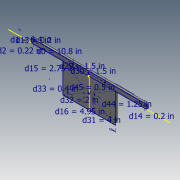
# Autodesk Inventor part: VP TRAY PUSHER TOP
Saved by Autodesk Inventor 2018.3 (Build 223284000, 284)
## iProperties
Created: 2019-10-29
Material: Generic
Vendor: HHMI: JRC - ID&F
Document SubType Name: Modeling
Designer: arnoldj
Density: 1 g/cm^3
Appearance: Default
RuleStatus: InUse
AfterDocSave0: file://Part Number Cleaner
DESIGN DEPARTMENT: HHMI: JRC - ID&F
ALTERED ITEM PART NUMBER: N/A
ALTERED ITEM VENDOR: N/A
ALTERED ITEM DESCRIPTION: N/A
Author: arnoldj
Revision Number: 0
Autodesk Inventor part; units mm, degrees
ref_plane "YZ Plane" through (0, 0, 0) normal (1, 0, 0) x (0, 1, 0)
ref_plane "XZ Plane" through (0, 0, 0) normal (0, 1, 0) x (-1, 0, 0)
ref_plane "XY Plane" through (0, 0, 0) normal (0, 0, 1) x (1, 0, 0)
sketch "Sketch1" plane through (0, 0, 0) normal (0, 0, 1) x (1, 0, 0)
  line L0 (0, 26.162) -> (0, -85.852) projected
  line L1 (-192.024, 0) -> (192.024, 0) projected
  line L2 (137.16, 10.16) -> (-137.16, 10.16)
  line L3 (-137.16, 10.16) -> (-137.16, 0)
  line L4 (-137.16, 0) -> (137.16, 0)
  line L5 (137.16, 0) -> (137.16, 10.16)
  line L6 (137.16, 10.16) -> (-137.16, 0) construction
  line L7 (-137.16, 10.16) -> (137.16, 0) construction
  line L8 (62.865, -69.85) -> (-62.865, -69.85)
  line L9 (-62.865, -69.85) -> (-62.865, 0)
  line L10 (-62.865, 0) -> (62.865, 0)
  line L11 (62.865, 0) -> (62.865, -69.85)
  line L12 (62.865, -69.85) -> (-62.865, 0) construction
  line L13 (-62.865, -69.85) -> (62.865, 0) construction
  point P0 (0, 0)
  point P1 (0, 5.08)
  point P2 (0, 5.588)
  point P3 (-132.08, 5.588)
  point P4 (132.08, 5.588)
  point P5 (0, -34.925)
  point P6 (12.7, -31.75)
  point P7 (-38.1, 5.588)
  point P8 (38.1, 5.588)
  point P9 (-50.8, -59.69)
  point P10 (50.8, -59.69)
  point P11 (0, -34.925)
  dimension "d0" = 274.32
  dimension "d1" = 10.16
  dimension "d2" = 5.588
  dimension "d13" = 5.08
  dimension "d14" = 5.08
  dimension "d15" = 69.85
  dimension "d16" = 125.73
  dimension "d29" = 38.1
  dimension "d30" = 38.1
  dimension "d31" = 101.6
  dimension "d32" = 50.8
  dimension "d33" = 10.16
  dimension "d44" = 31.75
  dimension "d45" = 12.7
  constraints: 24 end point, 5 midpoint, 5 point on line, 4 parallel, 2 horizontal, 2 horizontal alignment, 2 perpendicular
  measures "d0" distance of L2.start L2.end
  measures "d1" distance of L2.end L3.end
  measures "d2" distance from line of L4 point (-132.08, 5.588)
  measures "d13" distance from line of point (-132.08, 5.588) L3
  measures "d14" distance from line of L5 point (132.08, 5.588)
  measures "d15" distance of L8.end L9.end
  measures "d16" distance of L8.start L8.end
  measures "d29" distance of point (0, 5.588) point (-38.1, 5.588)
  measures "d30" distance of point (0, 5.588) point (38.1, 5.588)
  measures "d31" distance of point (50.8, -59.69) point (-50.8, -59.69)
  measures "d32" distance from line of L0 point (-50.8, -59.69)
  measures "d33" distance from line of L8 point (-50.8, -59.69)
  measures "d44" distance from line of L1 point (12.7, -31.75)
  measures "d45" distance from line of L0 point (12.7, -31.75)
extrude "Extrusion1" add sketch "Sketch1" against normal blind 4.4958 contours L2 L5 L1 L0 | L0 L1 L3 L2
hole "Hole1" at (0, 5.588, 0) at (-132.08, 5.588, 0) at (132.08, 5.588, 0) at (-38.1, 5.588, 0) at (38.1, 5.588, 0) direction (0, 0, -1) diameter 3.81 end through all clearance for "Socket Head Cap Screw" size "#6" standard "Ansi Unified Screw Threads"
fillet "Fillet1" radius 3.175 2 edges at (-137.16, 10.16, -2.2479) (137.16, 10.16, -2.2479)
extrude "Extrusion2" add sketch "Sketch1" against normal up to surface (4.4958 mm away) contours L1 L11 L8 L0 | L0 L8 L9 L1
fillet "Fillet2" radius 9.525 2 edges at (-62.865, -69.85, -2.2479) (62.865, -69.85, -2.2479)
hole "Hole2" at (12.7, -31.75, 0) direction (0, 0, -1) diameter 3.3528 end through all
hole "Hole3" at (-50.8, -59.69, 0) at (50.8, -59.69, 0) direction (0, 0, -1) diameter 3.81 end through all clearance for "Socket Head Cap Screw" size "#6" standard "Ansi Unified Screw Threads"
pattern_linear "Rectangular Pattern1" count 4 spacing 9.525 along (0, -1, 0) count 2 spacing 25.4 along (-1, 0, 0) of "Hole2"
body "Solid1"
